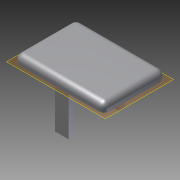
# Autodesk Inventor part: GearBoxTop
Saved by Autodesk Inventor 2012 (Build 160160000, 160)
## iProperties
Created: 2011-10-22
Part Number: GearBoxTop
Material: Default
Document SubType Name: Modeling
Designer: KuttaA
Density: 1 g/cm^3
Author: KuttaA
Autodesk Inventor part; units mm, degrees
ref_plane "YZ Plane" through (0, 0, 0) normal (1, 0, 0) x (0, 1, 0)
ref_plane "XZ Plane" through (0, 0, 0) normal (0, 1, 0) x (-1, 0, 0)
sketch "Sketch1" plane through (0, 0, 0) normal (0, 0, 1) x (1, 0, 0)
  arc A0 (-31.9035, -17) -> (-29.9035, -19) centre (-29.9035, -17) ccw projected
  line L0 (-29.9035, -19) -> (-2, -19) projected
  arc A1 (-2, -19) -> (0, -17) centre (-2, -17) ccw projected
  line L1 (0, 1) -> (0, -17) projected
  arc A2 (0, 1) -> (-2, 3) centre (-2, 1) ccw projected
  line L2 (-2, 3) -> (-29.9035, 3) projected
  arc A3 (-29.9035, 3) -> (-31.9035, 1) centre (-29.9035, 1) ccw projected
  line L3 (-31.9035, -17) -> (-31.9035, 1) projected
  line L4 (-17.2029, -18.3) -> (-17.2029, -16) projected
  line L5 (-28.9035, -16) -> (-17.2029, -16) projected
  line L6 (-28.9035, 0) -> (-28.9035, -16) projected
  line L7 (-17.2029, 0) -> (-28.9035, 0) projected
  line L8 (-17.2029, 0) -> (-17.2029, 2.3) projected
  line L9 (-17.2029, 2.3) -> (-14.6938, 2.3) projected
  line L10 (-14.6938, 2.3) -> (-14.6938, 0) projected
  line L11 (-3, 0) -> (-14.6938, 0) projected
  line L12 (-3, 0) -> (-3, -16) projected
  line L13 (-14.6938, -16) -> (-3, -16) projected
  line L14 (-14.6938, -16) -> (-14.6938, -18.3) projected
  line L15 (-17.2029, -18.3) -> (-14.6938, -18.3) projected
  line L16 (-14.6938, -16) -> (-17.2029, -16)
  line L17 (-14.6938, 0) -> (-17.2029, 0)
  line L18 (-16.9029, -16) -> (-14.9938, -16)
  line L19 (-14.9938, -16) -> (-14.9938, -18)
  line L20 (-14.9938, -18) -> (-16.9029, -18)
  line L21 (-16.9029, -18) -> (-16.9029, -16)
  line L22 (-16.9029, 2) -> (-14.9938, 2)
  line L23 (-14.9938, 2) -> (-14.9938, 0)
  line L24 (-14.9938, 0) -> (-16.9029, 0)
  line L25 (-16.9029, 0) -> (-16.9029, 2)
  point P0 (0, 0)
  dimension "d5" = 0.3
  dimension "d6" = 0
  dimension "d7" = 0.3
  dimension "d8" = 0.3
  dimension "d9" = 0.3
  dimension "d10" = 0.3
  dimension "d11" = 0.3
  dimension "d12" = 0
  constraints: 20 end point, 6 parallel, 2 horizontal, 2 perpendicular
  measures "d5" distance between parallel lines of L15 L20
  measures "d6" distance between parallel lines of L16 L18
  measures "d7" distance between parallel lines of L14 L19
  measures "d8" distance between parallel lines of L4 L21
  measures "d9" distance between parallel lines of L9 L22
  measures "d10" distance between parallel lines of L10 L23
  measures "d11" distance between parallel lines of L8 L25
  measures "d12" distance between parallel lines of L24 L17
extrude "Extrusion1" add sketch "Sketch1" against normal blind 14.9 contours L16 L19 L20 L21 | L25 L22 L23 L17
ref_plane "Work Plane1" through (0, 0, 0) normal (0, 0, 1) x (1, 0, 0)
sketch "Sketch2" plane through (0, 0, 0) normal (0, 0, 1) x (1, 0, 0)
  arc A0 (-31.9035, -17) -> (-29.9035, -19) centre (-29.9035, -17) ccw projected
  line L0 (-29.9035, -19) -> (-2, -19) projected
  arc A1 (-2, -19) -> (0, -17) centre (-2, -17) ccw projected
  line L1 (0, 1) -> (0, -17) projected
  arc A2 (0, 1) -> (-2, 3) centre (-2, 1) ccw projected
  line L2 (-2, 3) -> (-29.9035, 3) projected
  arc A3 (-29.9035, 3) -> (-31.9035, 1) centre (-29.9035, 1) ccw projected
  line L3 (-31.9035, -17) -> (-31.9035, 1) projected
  line L4 (-17.2029, -18.3) -> (-17.2029, -16) projected
  line L5 (-28.9035, -16) -> (-17.2029, -16) projected
  line L6 (-28.9035, 0) -> (-28.9035, -16) projected
  line L7 (-17.2029, 0) -> (-28.9035, 0) projected
  line L8 (-17.2029, 0) -> (-17.2029, 2.3) projected
  line L9 (-17.2029, 2.3) -> (-14.6938, 2.3) projected
  line L10 (-14.6938, 2.3) -> (-14.6938, 0) projected
  line L11 (-3, 0) -> (-14.6938, 0) projected
  line L12 (-3, 0) -> (-3, -16) projected
  line L13 (-14.6938, -16) -> (-3, -16) projected
  line L14 (-14.6938, -16) -> (-14.6938, -18.3) projected
  line L15 (-17.2029, -18.3) -> (-14.6938, -18.3) projected
  line L16 (-17.2029, 0) -> (-14.6938, 0) projected
  line L17 (-14.6938, 0) -> (-14.6938, 2.3) projected
  line L18 (-14.6938, 2.3) -> (-17.2029, 2.3) projected
  line L19 (-17.2029, 2.3) -> (-17.2029, 0) projected
  line L20 (-17.2029, -18.3) -> (-14.6938, -18.3) projected
  line L21 (-14.6938, -18.3) -> (-14.6938, -16) projected
  line L22 (-14.6938, -16) -> (-17.2029, -16) projected
  line L23 (-17.2029, -16) -> (-17.2029, -18.3) projected
  point P0 (0, 0)
extrude "Extrusion2" add sketch "Sketch2" along normal blind 3 contours L3 A3 L2 A2 L1 A1 L0 A0 | L4 L22 L14 L15 | L5 L6 L7 L16 L11 L12 L13 L22 | L8 L9 L10 L16
fillet "Fillet1" radius 2 8 edges at (-31.3177, -18.4142, 3) (-31.9035, -8, 3) (-31.3177, 2.4142, 3) (-15.9518, 3, 3) (-0.5858, 2.4142, 3) (0, -8, 3) (-0.5858, -18.4142, 3) (-15.9518, -19, 3)
sketch "Sketch3" plane through (0, 0, 0) normal (0, 0, -1) x (-1, 0, 0)
  arc A0 (29.9035, -19) -> (31.9035, -17) centre (29.9035, -17) ccw projected
  line L0 (29.9035, -19) -> (2, -19) projected
  arc A1 (0, -17) -> (2, -19) centre (2, -17) ccw projected
  line L1 (0, 1) -> (0, -17) projected
  arc A2 (2, 3) -> (0, 1) centre (2, 1) ccw projected
  line L2 (2, 3) -> (29.9035, 3) projected
  arc A3 (31.9035, 1) -> (29.9035, 3) centre (29.9035, 1) ccw projected
  line L3 (31.9035, -17) -> (31.9035, 1) projected
  line L4 (17.2029, -18.3) -> (17.2029, -16) projected
  line L5 (28.9035, -16) -> (17.2029, -16) projected
  line L6 (28.9035, 0) -> (28.9035, -16) projected
  line L7 (17.2029, 0) -> (28.9035, 0) projected
  line L8 (17.2029, 0) -> (17.2029, 2.3) projected
  line L9 (17.2029, 2.3) -> (14.6938, 2.3) projected
  line L10 (14.6938, 2.3) -> (14.6938, 0) projected
  line L11 (3, 0) -> (14.6938, 0) projected
  line L12 (3, 0) -> (3, -16) projected
  line L13 (14.6938, -16) -> (3, -16) projected
  line L14 (14.6938, -16) -> (14.6938, -18.3) projected
  line L15 (17.2029, -18.3) -> (14.6938, -18.3) projected
  line L16 (14.9938, 0) -> (16.9029, 0) projected
  line L17 (14.9938, 0) -> (14.9938, -0.3)
  line L18 (14.9938, -0.3) -> (3.3, -0.3)
  line L19 (3.3, -0.3) -> (3.3, -1.8)
  line L20 (3.3, -1.8) -> (28.6035, -1.8)
  line L21 (28.6035, -0.3) -> (16.9029, -0.3)
  line L22 (16.9029, 0) -> (16.9029, -0.3)
  line L23 (28.6035, -1.8) -> (28.6035, -0.3)
  line L24 (3, -8) -> (28.9035, -8) construction
  line L25 (14.9938, -16) -> (16.9029, -16)
  line L26 (14.9938, -16) -> (14.9938, -15.7)
  line L27 (14.9938, -15.7) -> (3.3, -15.7)
  line L28 (3.3, -15.7) -> (3.3, -14.2)
  line L29 (3.3, -14.2) -> (28.6035, -14.2)
  line L30 (28.6035, -15.7) -> (16.9029, -15.7)
  line L31 (16.9029, -16) -> (16.9029, -15.7)
  line L32 (28.6035, -14.2) -> (28.6035, -15.7)
  line L33 (3.3, -1.8) -> (3.3, -14.2)
  line L34 (4.8, -14.2) -> (4.8, -1.8)
  line L35 (28.6035, -1.8) -> (28.6035, -14.2)
  line L36 (27.1035, -14.2) -> (27.1035, -1.8)
  point P0 (0, 0)
  dimension "d13" = 0.3
  dimension "d14" = 0.3
  dimension "d15" = 1.5
  dimension "d16" = 0.3
  dimension "d17" = 0.3
  dimension "d20" = 1.5
  dimension "d21" = 1.5
  constraints: 40 end point, 8 symmetric about line, 6 parallel, 5 perpendicular, 4 point on line, 2 midpoint
  measures "d13" distance between parallel lines of L7 L21
  measures "d14" distance between parallel lines of L11 L18
  measures "d15" distance between parallel lines of L18 L20
  measures "d16" distance between parallel lines of L12 L19
  measures "d17" distance between parallel lines of L6 L23
  measures "d20" distance between parallel lines of L33 L34
  measures "d21" distance between parallel lines of L35 L36
extrude "Extrusion3" add sketch "Sketch3" along normal blind 3 contours L16 L22 L21 L23 L20 L19 L18 L17 | L20 L34 L29 L33 | L35 L29 L36 L20 | L29 L32 L30 L31 L25 L26 L27 L28
sketch "Sketch4" plane through (-14.9938, -18, -14.9) normal (1, 0, 0) x (0, 0, -1)
  line L0 (-14.9, -0.3) -> (2.2893, -0.3) projected
  line L1 (-14.9, 2) -> (-14.9, -0.3) projected
  line L2 (2.2893, 2) -> (-14.9, 2) projected
  line L3 (2.2893, 2) -> (2.2893, -0.3) projected
  line L4 (0, 2) -> (0, 0) projected
  line L5 (-14.9, 0) -> (0, 0) projected
  line L6 (-14.9, 2.3) -> (-14.9, 0) projected
  line L7 (-14.9, 2.3) -> (-11.9, 2.3) projected
  line L8 (-11.9, 2.3) -> (-11.9, 2) projected
  line L9 (-11.9, 2) -> (0, 2) projected
  line L10 (0, 18) -> (0, 20) projected
  line L11 (-14.9, 20) -> (0, 20) projected
  line L12 (-14.9, 20) -> (-14.9, 17.7) projected
  line L13 (-14.9, 17.7) -> (-11.9, 17.7) projected
  line L14 (-11.9, 17.7) -> (-11.9, 18) projected
  line L15 (-11.9, 18) -> (0, 18) projected
  line L16 (-7.45, 2) -> (-11.9, 4.6913)
  line L17 (-11.9, 4.6913) -> (-11.9, 2.3)
  line L18 (-11.9, 10) -> (3.9744, 10) construction
  line L19 (-7.45, 18) -> (-11.9, 15.3087)
  line L20 (-11.9, 15.3087) -> (-11.9, 17.7)
  point P0 (-14.9, 18)
  constraints: 10 end point, 2 point on line, 2 symmetric about line, 1 perpendicular
extrude "Extrusion4" add sketch "Sketch4" against normal up to surface (1.9092 mm away) contours L8 L17 L16 L2 | L19 L20 L14 L15
sketch "Sketch6" plane through (0, 0, 0) normal (0, 0, -1) x (-1, 0, 0)
  line L0 (27.1035, -1.8) -> (4.8, -1.8) projected
  line L1 (4.8, -1.8) -> (4.8, -14.2) projected
  line L2 (4.8, -14.2) -> (27.1035, -14.2) projected
  line L3 (27.1035, -14.2) -> (27.1035, -1.8) projected
  line L4 (14.9938, -13.3087) -> (16.9029, -13.3087) projected
  line L5 (14.9938, -2.6913) -> (16.9029, -2.6913) projected
  line L6 (14.9938, -2.6913) -> (5.6913, -2.6913)
  line L7 (5.6913, -2.6913) -> (5.6913, -13.3087)
  line L8 (5.6913, -13.3087) -> (14.9938, -13.3087)
  line L9 (16.9029, -13.3087) -> (26.2122, -13.3087)
  line L10 (26.2122, -13.3087) -> (26.2122, -2.6913)
  line L11 (26.2122, -2.6913) -> (16.9029, -2.6913)
  point P0 (0, 0)
  dimension "d24" = 0.8913
  dimension "d25" = 0.8913
  dimension "d26" = 0.8913
  constraints: 12 end point, 3 parallel, 2 perpendicular, 1 collinear
  measures "d24" distance between parallel lines of L0 L5
  measures "d25" distance between parallel lines of L1 L7
  measures "d26" distance between parallel lines of L3 L10
extrude "Extrusion5" add sketch "Sketch6" along normal up to surface (3 mm away)
sketch "Sketch7" plane through (0, 0, 0) normal (0, 0, -1) x (-1, 0, 0)
  line L0 (14.9938, -2.6913) -> (14.9938, -0.3) projected
  line L1 (3.3, -0.3) -> (14.9938, -0.3) projected
  line L2 (3.3, -15.7) -> (3.3, -0.3) projected
  line L3 (14.9938, -15.7) -> (3.3, -15.7) projected
  line L4 (14.9938, -13.3087) -> (14.9938, -15.7) projected
  line L5 (5.6913, -13.3087) -> (14.9938, -13.3087) projected
  line L6 (5.6913, -2.6913) -> (5.6913, -13.3087) projected
  line L7 (14.9938, -2.6913) -> (5.6913, -2.6913) projected
  line L8 (16.9029, -0.3) -> (16.9029, -2.6913) projected
  line L9 (26.2122, -2.6913) -> (16.9029, -2.6913) projected
  line L10 (26.2122, -13.3087) -> (26.2122, -2.6913) projected
  line L11 (16.9029, -13.3087) -> (26.2122, -13.3087) projected
  line L12 (16.9029, -13.3087) -> (16.9029, -15.7) projected
  line L13 (28.6035, -15.7) -> (16.9029, -15.7) projected
  line L14 (28.6035, -0.3) -> (28.6035, -15.7) projected
  line L15 (16.9029, -0.3) -> (28.6035, -0.3) projected
  line L16 (5.6913, -8) -> (10.3425, -13.3087)
  line L17 (5.6913, -8) -> (10.3425, -2.6913)
  line L18 (21.5576, -2.6913) -> (26.2122, -8)
  line L19 (26.2122, -8) -> (21.5576, -13.3087)
  point P0 (0, 0)
  constraints: 8 end point, 6 midpoint
extrude "Extrusion6" add sketch "Sketch7" along normal up to surface (3 mm away) contours L17 L6 L7 | L16 L5 L6 | L9 L10 L18 | L10 L11 L19
sketch "Sketch8" plane through (0, 0, -14.9) normal (0, 0, -1) x (-1, 0, 0)
  line L0 (16.9029, 2) -> (16.9029, 0) projected
  line L1 (14.9938, 0) -> (14.9938, 2) projected
  line L2 (16.9029, 0) -> (14.9938, 0) projected
  line L3 (13.4938, 2) -> (18.4028, 2)
  line L4 (18.4028, 2) -> (18.4028, 0)
  line L5 (18.4028, 0) -> (13.4938, 0)
  line L6 (13.4938, 0) -> (13.4938, 2)
  line L7 (3.3, -15.7) -> (3.3, -0.3) projected
  line L8 (28.6035, -0.3) -> (28.6035, -15.7) projected
  line L9 (3.3, -8) -> (28.6035, -8) construction
  line L10 (13.4938, -18) -> (18.4028, -18)
  line L11 (18.4028, -18) -> (18.4028, -16)
  line L12 (18.4028, -16) -> (13.4938, -16)
  line L13 (13.4938, -16) -> (13.4938, -18)
  point P0 (0, 0)
  dimension "d31" = 4.909
  dimension "d32" = 1.9092
  dimension "d33" = 1.4999
  dimension "d34" = 0
  dimension "d35" = 2
  dimension "d36" = 2
  constraints: 18 end point, 4 symmetric about line, 2 midpoint, 2 parallel, 1 horizontal, 1 perpendicular
  measures "d31" distance of L3.start L3.end
  measures "d32" distance between parallel lines of L1 L0
  measures "d33" distance between parallel lines of L4 L0
  measures "d34" distance between parallel lines of L2 L5
  measures "d35" distance between parallel lines of L2 L3
  measures "d36" distance of L0.start L0.end
extrude "Extrusion7" add sketch "Sketch8" against normal up to surface (14.9 mm away)
sketch "Sketch9" plane through (-14.9938, -16, 0) normal (1, 0, 0) x (0, 0, -1)
  line L0 (0, 0) -> (7.45, 0) projected
  line L1 (7.45, 0) -> (3, 2.6913) projected
  line L2 (3, 2.6913) -> (3, 0.3) projected
  line L3 (0, 0.3) -> (3, 0.3) projected
  line L4 (0, 0) -> (0, 0.3) projected
  line L5 (7.45, 16) -> (0, 16) projected
  line L6 (0, 16) -> (0, 15.7) projected
  line L7 (0, 15.7) -> (3, 15.7) projected
  line L8 (3, 13.3087) -> (3, 15.7) projected
  line L9 (3, 13.3087) -> (7.45, 16) projected
  point P0 (0, 16)
extrude "Extrusion8" add sketch "Sketch9" along normal up to surface (1.4999 mm away)
sketch "Sketch10" plane through (-16.9029, -16, 0) normal (-1, 0, 0) x (0, 0, 1)
  line L0 (-7.45, 0) -> (0, 0) projected
  line L1 (0, 0.3) -> (0, 0) projected
  line L2 (0, 0.3) -> (-3, 0.3) projected
  line L3 (-3, 2.6913) -> (-3, 0.3) projected
  line L4 (-7.45, 0) -> (-3, 2.6913) projected
  line L5 (0, 16) -> (-7.45, 16) projected
  line L6 (-3, 13.3087) -> (-7.45, 16) projected
  line L7 (-3, 15.7) -> (-3, 13.3087) projected
  line L8 (0, 15.7) -> (-3, 15.7) projected
  line L9 (0, 16) -> (0, 15.7) projected
  point P0 (0, 16)
extrude "Extrusion9" add sketch "Sketch10" along normal up to surface (1.4999 mm away)
sketch "Sketch11" plane through (-21.5576, -2.6913, 0) normal (0, -1, 0) x (1, 0, 0)
  line L0 (11.2151, -3) -> (11.2151, 0) projected
  line L1 (0, 0) -> (11.2151, 0) projected
  line L2 (0, 0) -> (0, -3) projected
  line L3 (0, -3) -> (3.1547, -3) projected
  line L4 (3.1547, -3) -> (8.0637, -3) projected
  line L5 (8.0637, -3) -> (11.2151, -3) projected
  line L6 (8.0637, -7.45) -> (3.1547, -7.45) projected
  line L7 (3.1547, -3) -> (3.1547, -7.45) projected
  line L8 (8.0637, -7.45) -> (8.0637, -3) projected
  point P0 (21.5576, 0)
extrude "Extrusion10" cut sketch "Sketch11" against normal blind 0.4
sketch "Sketch12" plane through (-21.5576, -13.3087, 0) normal (0, 1, 0) x (1, 0, 0)
  line L0 (11.2151, 0) -> (11.2151, 3) projected
  line L1 (11.2151, 3) -> (8.0637, 3) projected
  line L2 (8.0637, 3) -> (3.1547, 3) projected
  line L3 (3.1547, 3) -> (0, 3) projected
  line L4 (0, 3) -> (0, 0) projected
  line L5 (11.2151, 0) -> (0, 0) projected
  line L6 (8.0637, 3.6614) -> (3.1547, 3.6614) projected
  line L7 (3.1547, 3.6614) -> (3.1547, 3) projected
  line L8 (8.0637, 3.6614) -> (8.0637, 3)
  point P0 (21.5576, 0)
  constraints: 2 end point, 1 parallel
extrude "Extrusion11" cut sketch "Sketch12" against normal blind 0.4
sketch "Sketch13" plane through (-18.4028, 0, -7.45) normal (0, -1, 0) x (1, 0, 0)
  line L0 (4.909, 0) -> (0, 0) projected
  line L1 (0, -7.45) -> (0, 0) projected
  line L2 (0, -7.45) -> (4.909, -7.45) projected
  line L3 (4.909, -7.45) -> (4.909, 0) projected
  point P0 (18.4028, 7.45)
ref_plane "Work Plane2" through (-20.3233, -0.3, -20.2296) normal (0, 1, 0) x (0, 0, 1)
extrude "Extrusion12" add sketch "Sketch13" along normal up to surface (0.3 mm away)
sketch "Sketch14" plane through (-18.4028, 2, -14.9) normal (0, 1, 0) x (1, 0, 0)
  line L0 (4.909, 0) -> (0, 0) projected
  line L1 (0, 0) -> (0, -14.9) projected
  line L2 (6.8295, -3.4204) -> (-1.9205, -3.4204)
  line L3 (0, -3.4204) -> (4.909, -3.4204)
  line L4 (4.909, -3.4204) -> (4.909, 0)
  line L5 (4.909, 0) -> (0, 0)
  line L6 (0, 0) -> (0, -3.4204)
  point P0 (18.4028, -14.9)
  constraints: 10 end point, 2 horizontal, 2 parallel, 2 point on line, 1 perpendicular, 2 other
extrude "Extrusion13" cut sketch "Sketch14" against normal up to surface (20 mm away)
ref_plane "Work Plane3" through (-20.3233, -0.3, -11.4796) normal (0, 0, 1) x (-1, 0, 0)
sketch "Sketch15" plane through (-20.3233, -0.3, -11.4796) normal (0, 0, 1) x (-1, 0, 0)
  line L0 (-8.75, 17.6961) -> (-8.75, 13)
  line L1 (0, 17.6961) -> (-8.75, 17.6961)
  line L2 (-8.75, 13) -> (0, 13)
  line L3 (0, 17.6961) -> (0, 13)
  line L4 (-8.75, 2.4) -> (-8.75, -2.3)
  line L5 (0, 2.4) -> (-8.75, 2.4)
  line L6 (-8.75, -2.3) -> (0, -2.3)
  line L7 (0, -2.3) -> (0, 2.4)
  point P0 (-20.3233, -0.3)
  constraints: 16 end point, 4 horizontal, 4 vertical, 8 other
extrude "Extrusion14" add sketch "Sketch15" along normal up to surface (11.4796 mm away)
equation "\"d7\" = d5"
equation "\"d8\" = d5"
equation "\"d9\" = d5"
equation "\"d10\" = d9"
equation "\"d11\" = d10"
equation "\"d20\" = d15"
equation "\"d21\" = d20"
equation "\"d25\" = d24"
equation "\"d26\" = d24"
equation "\"d33\" = -0.5 * d32 + 0.5 * d31"
equation "\"d35\" = d36"
body "Solid1"
